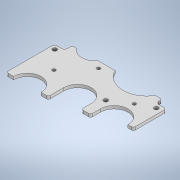
# Autodesk Inventor part: Bottle clamping plate 2
Saved by Autodesk Inventor 2021 (Build 250183000, 183)
## iProperties
Created: 2020-07-28
Part Number: Bottle clamping plate 2
Material: Generic
Document SubType Name: Modeling
Designer: jgray
Density: 1 g/cm^3
Appearance: Default
Author: jgray
Autodesk Inventor part; units mm, degrees
ref_plane "YZ Plane" through (0, 0, 0) normal (1, 0, 0) x (0, 1, 0)
ref_plane "XZ Plane" through (0, 0, 0) normal (0, 1, 0) x (-1, 0, 0)
ref_plane "XY Plane" through (0, 0, 0) normal (0, 0, 1) x (1, 0, 0)
sketch "Sketch1" plane through (0, 0, 0) normal (0, 1, 0) x (-1, 0, 0)
  line L0 (-56.25, 58.25) -> (56.25, 58.25)
  line L1 (56.25, 58.25) -> (56.25, -58.25)
  line L2 (56.25, -58.25) -> (-56.25, -58.25)
  line L3 (-56.25, -58.25) -> (-56.25, 58.25)
  line L4 (-56.25, 58.25) -> (56.25, -58.25) construction
  line L5 (56.25, 58.25) -> (-56.25, -58.25) construction
  point P0 (0, 0)
  dimension "d0" = 112.5
  dimension "d1" = 116.5
  constraints: 12 end point, 2 midpoint, 2 parallel, 1 horizontal, 1 perpendicular
  measures "d0" distance of L1.end L2.end
  measures "d1" distance of L0.end L1.end
extrude "Extrusion1" add sketch "Sketch1" along normal blind 3
sketch "Sketch2" plane through (0, 3, 0) normal (0, 1, 0) x (1, 0, 0)
  circle A0 centre (18.5, 28) radius 23.85
  circle A1 centre (37, -23.25) radius 13.85
  circle A2 centre (-35, -38.75) radius 13.85
  circle A3 centre (-30.9, 25.8) radius 13.85
  circle A4 centre (0, -23.25) radius 13.85
  line L0 (56.25, 58.25) -> (-56.25, 58.25) projected
  line L1 (-56.25, -58.25) -> (56.25, -58.25) projected
  line L2 (0, -105.9299) -> (0, 123.2086) construction
  line L3 (-76.4777, -38.75) -> (-5.35, -38.75) construction
  line L4 (-123.5447, -23.25) -> (82.5572, -23.25) construction
  line L5 (56.25, -58.25) -> (56.25, 58.25) construction
  point P0 (0, 0)
  dimension "d4" = 47.7
  dimension "d5" = 27.7
  dimension "d6" = 27.7
  dimension "d7" = 27.7
  dimension "d8" = 27.7
  dimension "d9" = 116.5
  dimension "d10" = 112.5
  dimension "d13" = 37
  dimension "d14" = 18.5
  dimension "d15" = 30.9
  dimension "d18" = 19.5
  dimension "d19" = 35
  dimension "d20" = 35
  dimension "d57" = 25.8
  dimension "d58" = 28
  dimension "d59" = 23.25
  constraints: 6 end point, 5 centre point, 5 point on line, 1 horizontal, 1 perpendicular, 1 vertical
  measures "d4" diameter of A0
  measures "d5" diameter of A1
  measures "d6" diameter of A2
  measures "d7" diameter of A3
  measures "d8" diameter of A4
  measures "d9" distance between parallel lines of L0 L1
  measures "d10" distance of L1.start L1.end
  measures "d13" distance of A4.centre A1.centre
  measures "d14" distance from line of A0.centre L2
  measures "d15" distance from line of A3.centre L2
  measures "d18" distance between parallel lines of L1 L3
  measures "d19" distance between parallel lines of L1 L4
  measures "d20" horizontal distance of A2.centre A4.centre
  measures "d57" vertical distance of point (0, 0) A3.centre
  measures "d58" vertical distance of point (0, 0) A0.centre
  measures "d59" distance from line of point (0, 0) L4
extrude "Extrusion2" cut sketch "Sketch2" against normal blind 5
sketch "Sketch3" plane through (0, 3, 0) normal (0, 1, 0) x (1, 0, 0)
  line L0 (-56.25, 58.25) -> (-56.25, -58.25)
  line L1 (56.25, -58.25) -> (56.25, 58.25)
  line L2 (18.5, -17.4904) -> (18.5, -40.0394) construction
  line L3 (-51.55, 5.4) -> (-51.55, 71.9941) construction
  line L4 (50.75, 5.4) -> (50.75, 69.4565) construction
  line L5 (-73.722, 50) -> (66.5467, 50) construction
  line L6 (66.5467, 30) -> (-76.0779, 30) construction
  circle A0 centre (18.5, 28) radius 23.85 projected
  circle A1 centre (37, -23.25) radius 13.85 projected
  circle A2 centre (-30.9, 25.8) radius 13.85 projected
  circle A3 centre (0, -23.25) radius 13.85 projected
  circle A4 centre (-35, -38.75) radius 13.85 projected
  line L7 (56.25, 58.25) -> (-56.25, 58.25) projected
  line L8 (-56.25, 58.25) -> (-56.25, -58.25) projected
  line L9 (-56.25, -58.25) -> (56.25, -58.25) projected
  line L10 (56.25, -58.25) -> (56.25, 58.25) projected
  circle A5 centre (-30.9, 25.8) radius 13.85
  circle A6 centre (18.5, 28) radius 23.85
  circle A7 centre (0, -23.25) radius 13.85
  circle A8 centre (37, -23.25) radius 13.85
  circle A9 centre (-35, -38.75) radius 13.85
  line L11 (-56.25, 58.25) -> (-56.25, -58.25) projected
  line L12 (-56.25, 58.25) -> (-56.25, -58.25)
  line L13 (56.25, -58.25) -> (56.25, 58.25) projected
  line L14 (56.25, 58.25) -> (56.25, -58.25)
  line L15 (-56.25, 17.5) -> (-41.9875, 17.5)
  line L16 (-19.8125, 17.5) -> (-2.9143, 17.5)
  line L17 (39.1112, 16) -> (56.25, 16)
  line L18 (-56.25, -38.75) -> (-48.85, -38.75)
  circle A10 centre (-35, -38.75) radius 13.85 projected
  circle A11 centre (37, -23.25) radius 13.85 projected
  line L19 (50.85, -23.25) -> (56.25, -23.25)
  circle A12 centre (0, -23.25) radius 13.85 projected
  line L20 (-13.85, -23.25) -> (-13.85, -36.75)
  line L21 (-15.85, -38.75) -> (-21.15, -38.75)
  line L22 (13.85, -23.25) -> (13.85, -31.25)
  line L23 (15.85, -33.25) -> (21.15, -33.25)
  line L24 (23.15, -31.25) -> (23.15, -23.25)
  arc A13 (13.85, -31.25) -> (15.85, -33.25) centre (15.85, -31.25) ccw
  arc A14 (21.15, -33.25) -> (23.15, -31.25) centre (21.15, -31.25) ccw
  arc A15 (-15.85, -38.75) -> (-13.85, -36.75) centre (-15.85, -36.75) ccw
  point P0 (0, 0)
  point P1 (0, 0)
  point P2 (18.5, -13.25)
  point P3 (18.5, -23.25)
  point P4 (-51.55, 50)
  point P5 (-51.55, 30)
  point P6 (50.75, 50)
  point P7 (50.75, 30)
  point P8 (-13.85, -38.75)
  point P9 (13.85, -33.25)
  point P10 (-2.9143, 17.5)
  point P11 (-56.25, -38.75)
  dimension "d21" = 4.7
  dimension "d22" = 5.5
  dimension "d23" = 13.25
  dimension "d24" = 30
  dimension "d25" = 50
  dimension "d26" = 5.4
  dimension "d27" = 5.4
  dimension "d29" = 18.5
  dimension "d31" = 10
  dimension "d32" = 2
  dimension "d55" = 27.7
  dimension "d56" = 47.7
  dimension "d60" = 2
  dimension "d61" = 27.7
  dimension "d62" = 23.25
  dimension "d63" = 37
  dimension "d64" = 17.5
  dimension "d65" = 17.5
  dimension "d66" = 16
  constraints: 38 end point, 23 point on line, 12 point on circle, 9 vertical, 7 centre point, 7 tangent, 6 coincident, 5 perpendicular, 3 horizontal alignment, 2 concentric, 2 horizontal, 2 line through centre, 2 parallel, 1 equal radius, 8 other
  measures "d21" distance from line of L0 L3.start
  measures "d22" distance from line of L1 L4.start
  measures "d23" vertical distance of point (0, 0) point (18.5, -13.25)
  measures "d24" distance from line of point (0, 0) L6
  measures "d25" distance from line of point (0, 0) L5
  measures "d26" vertical distance of point (0, 0) L4.start
  measures "d27" vertical distance of point (0, 0) L3.start
  measures "d29" distance from line of point (0, 0) L2
  measures "d31" distance of L22.start point (13.85, -33.25)
  measures "d32" radius of A13
  measures "d55" diameter of A5
  measures "d56" diameter of A0
  measures "d60" radius of A15
  measures "d61" diameter of A1
  measures "d62" vertical distance of point (0, 0) A1.centre
  measures "d63" horizontal distance of A1.centre point (0, 0)
  measures "d64" distance from line of point (0, 0) L15
  measures "d65" distance from line of point (0, 0) L16
  measures "d66" distance from line of point (0, 0) L17
hole "Hole1" at (-51.55, 3, -5.4) at (50.75, 3, -5.4) at (18.5, 3, 13.25) at (-51.55, 3, -50) at (-51.55, 3, -30) at (50.75, 3, -50) at (50.75, 3, -30) direction (0, -1, 0) diameter 4.2 end through all
extrude "Extrusion3" cut sketch "Sketch3" against normal blind 10 contours L7 L1 L17 A0 L16 A2 L15 L0 | L18 A4 L21 A15 L20 A3 L22 A13 L23 A14 L24 A1 L19 L1 L9 L0 | A3
sketch "Sketch4" plane through (0, 3, 0) normal (0, 1, 0) x (1, 0, 0)
  line L0 (-50.25, 75.9498) -> (-50.25, -88.0061) construction
  line L1 (-63.9145, -52.25) -> (79.4097, -52.25) construction
  line L2 (50.25, 66.2924) -> (50.25, -77.9097) construction
  line L3 (-56.25, 58.25) -> (-56.25, -58.25) construction
  line L4 (-56.25, -58.25) -> (56.25, -58.25) construction
  line L5 (56.25, -58.25) -> (56.25, 58.25) construction
  line L6 (-71.816, 40) -> (84.2384, 40) construction
  line L7 (-70.7185, 14) -> (79.4097, 14) construction
  line L8 (-56.25, 17.5) -> (-56.25, -38.75) projected
  line L9 (-56.25, 17.5) -> (-46.05, 17.5)
  line L10 (-46.05, 17.5) -> (-46.05, 12.8)
  line L11 (-49.05, 9.8) -> (-56.25, 9.8)
  line L12 (-56.25, 9.8) -> (-56.25, 17.5)
  line L13 (56.25, -23.25) -> (56.25, 16) projected
  line L14 (56.25, 16) -> (46.05, 16)
  line L15 (46.05, 16) -> (46.05, 12.8)
  line L16 (49.05, 9.8) -> (56.25, 9.8)
  line L17 (56.25, 9.8) -> (56.25, 16)
  line L18 (56.25, -23.25) -> (56.25, 16) projected
  line L19 (-56.25, 17.5) -> (-56.25, -38.75) projected
  arc A0 (-49.05, 9.8) -> (-46.05, 12.8) centre (-49.05, 12.8) ccw
  arc A1 (46.05, 12.8) -> (49.05, 9.8) centre (49.05, 12.8) ccw
  point P0 (0, 0)
  point P1 (0, 0)
  point P2 (-50.25, 40)
  point P3 (-50.25, 14)
  point P4 (-50.25, -52.25)
  point P5 (50.25, -52.25)
  point P6 (0, -52.25)
  point P7 (50.25, 14)
  point P8 (50.25, 40)
  dimension "d42" = 6
  dimension "d43" = 6
  dimension "d44" = 6
  dimension "d45" = 14
  dimension "d46" = 40
  dimension "d47" = 4.2
  dimension "d48" = 14
  dimension "d49" = 4.2
  dimension "d50" = 4.2
  dimension "d52" = 3
  constraints: 32 end point, 13 point on line, 5 horizontal, 4 parallel, 4 point on circle, 4 tangent, 3 collinear, 2 centre point, 2 perpendicular, 2 vertical, 1 equal radius
  measures "d42" distance between parallel lines of L3 L0
  measures "d43" distance between parallel lines of L4 L1
  measures "d44" distance between parallel lines of L5 L2
  measures "d45" distance from line of point (0, 0) L7
  measures "d46" distance from line of point (0, 0) L6
  measures "d47" distance between parallel lines of L10 L0
  measures "d48" distance from line of point (0, 0) L7
  measures "d49" distance between parallel lines of L11 L7
  measures "d50" distance between parallel lines of L15 L2
  measures "d52" radius of A0
extrude "Extrusion4" cut sketch "Sketch4" against normal blind 10
fillet "Fillet1" radius 2 4 edges at (-56.25, 1.5, 38.75) (56.25, 1.5, 23.25) (56.25, 1.5, -9.8) (-56.25, 1.5, -9.8)
sketch "Sketch5" plane through (0, 3, 0) normal (0, 1, 0) x (1, 0, 0)
  point P0 (0, 0)
  point P1 (0, 0)
  point P2 (-34, -13)
  point P3 (-13, 11)
  point P4 (36, -2)
  dimension "d68" = 13
  dimension "d69" = 34
  dimension "d70" = 36
  dimension "d71" = 2
  dimension "d72" = 11
  dimension "d73" = 13
  measures "d68" horizontal distance of point (-13, 11) point (0, 0)
  measures "d69" horizontal distance of point (-34, -13) point (0, 0)
  measures "d70" horizontal distance of point (36, -2) point (0, 0)
  measures "d71" vertical distance of point (36, -2) point (0, 0)
  measures "d72" vertical distance of point (-13, 11) point (0, 0)
  measures "d73" vertical distance of point (-34, -13) point (0, 0)
hole "Hole2" at (-34, 3, 13) at (-13, 3, -11) at (36, 3, 2) direction (0, -1, 0) diameter 3.2 end through all
fillet "Fillet2" radius 2 2 edges at (-46.05, 1.5, -17.5) (46.05, 1.5, -16)
body "Solid1"
